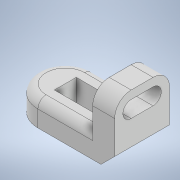
# Autodesk Inventor part: 1번부품
Saved by Autodesk Inventor 2022 (Build 260153000, 153)
## iProperties
Created: 2021-09-04
Part Number: 1번부품
Material: 일반
Document SubType Name: Modeling
Designer: 서울공업고등학교
Density: 1 g/cm^3
Appearance: 기본값
Author: 서울공업고등학교
Autodesk Inventor part; units mm, degrees
ref_plane "YZ Plane" through (0, 0, 0) normal (1, 0, 0) x (0, 1, 0)
ref_plane "XZ Plane" through (0, 0, 0) normal (0, 1, 0) x (-1, 0, 0)
ref_plane "XY Plane" through (0, 0, 0) normal (0, 0, 1) x (1, 0, 0)
sketch "스케치1" plane through (0, 0, 0) normal (0, 0, 1) x (1, 0, 0)
  line L0 (0, 0) -> (0, -9)
  line L1 (0, -9) -> (38, -9)
  line L2 (38, -9) -> (38, 14)
  line L3 (38, 14) -> (30, 14)
  line L4 (30, 14) -> (30, 0)
  line L5 (30, 0) -> (0, 0)
  dimension "d0" = 8
  dimension "d1" = 23
  dimension "d2" = 38
  dimension "d3" = 9
  constraints: 12 end point, 5 perpendicular, 1 vertical
  measures "d0" distance between parallel lines of L2 L4
  measures "d1" distance between parallel lines of L1 L3
  measures "d2" distance between parallel lines of L2 L0
  measures "d3" distance between parallel lines of L1 L5
extrude "돌출1" add sketch "스케치1" along normal mid plane 20
sketch "스케치2" plane through (38, -9, 10) normal (1, 0, 0) x (0, 0, -1)
  line L0 (6, 17) -> (14, 17) construction
  line L1 (6, 14) -> (14, 14)
  line L2 (14, 20) -> (6, 20)
  arc A0 (6, 20) -> (6, 14) centre (6, 17) ccw
  arc A1 (14, 14) -> (14, 20) centre (14, 17) ccw
  line L3 (20, 0) -> (0, 0) projected
  line L4 (0, 0) -> (0, 23) projected
  point P0 (10, 9)
  point P1 (10, 17)
  dimension "d7" = 8
  dimension "d8" = 6
  dimension "d9" = 3
  dimension "d10" = 17
  dimension "d11" = 10
  constraints: 8 end point, 4 point on circle, 4 tangent, 2 centre point, 1 horizontal, 1 midpoint, 1 parallel
  measures "d7" distance of L0.end L0.start
  measures "d8" distance between parallel lines of L1 L2
  measures "d9" radius of A0
  measures "d10" distance from line of L3 point (10, 17)
  measures "d11" distance from line of point (10, 17) L4
extrude "돌출2" cut sketch "스케치2" against normal blind 20
sketch "스케치3" plane through (0, 0, 10) normal (0, 1, 0) x (1, 0, 0)
  line L0 (10, 14) -> (30, 14)
  line L1 (30, 14) -> (30, 6)
  line L2 (30, 6) -> (10, 6)
  line L3 (10, 6) -> (10, 14)
  line L4 (0, 20) -> (0, 0) projected
  line L5 (30, 0) -> (0, 0) projected
  point P0 (0, 10)
  dimension "d14" = 8
  dimension "d15" = 20
  dimension "d16" = 10
  dimension "d17" = 6
  constraints: 8 end point, 2 parallel, 1 horizontal, 1 perpendicular
  measures "d14" distance between parallel lines of L2 L0
  measures "d15" distance of L0.start L0.end
  measures "d16" distance between parallel lines of L3 L4
  measures "d17" distance between parallel lines of L2 L5
extrude "돌출3" cut sketch "스케치3" against normal blind 20
chamfer "모따기1" distance 5 angle 45 1 edges at (38, -9, 0)
fillet "모깎기1" radius 10 2 edges at (0, -4.5, -10) (0, -4.5, 10)
fillet "모깎기2" radius 3 3 edges at (2.9289, 0, -7.0711) (20, 0, -10) (20, 0, 10)
fillet "모깎기3" radius 6 2 edges at (34, 14, 10) (34, 14, -10)
